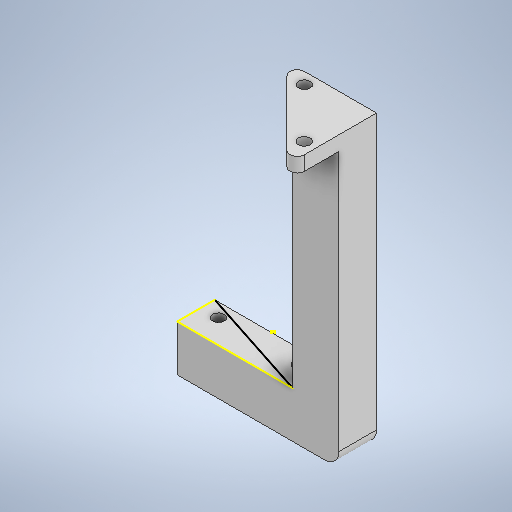
# Autodesk Inventor part: 13042026-12
Saved by Autodesk Inventor 2025.2 (Build 292293000, 293)
## iProperties
Created: 2026-05-05
Part Number: 13042026-12
Material: Generic
Document SubType Name: Modeling
Designer: Oski
Density: 1 g/cm^3
Appearance: Default
Author: Oski
Autodesk Inventor part; units mm, degrees
ref_plane "YZ Plane" through (0, 0, 0) normal (1, 0, 0) x (0, 1, 0)
ref_plane "XZ Plane" through (0, 0, 0) normal (0, 1, 0) x (-1, 0, 0)
ref_plane "XY Plane" through (0, 0, 0) normal (0, 0, 1) x (1, 0, 0)
sketch "Sketch2" plane through (0, 0, 0) normal (0, 0, 1) x (1, 0, 0)
  line L0 (-40, 16) -> (40, 16)
  line L1 (40, 16) -> (40, -16)
  line L2 (40, -16) -> (-40, -16)
  line L3 (-40, -16) -> (-40, 16)
  line L4 (-40, 16) -> (40, -16) construction
  line L5 (40, 16) -> (-40, -16) construction
  point P0 (0, 0)
  dimension "d4" = 32
  dimension "d5" = 80
  constraints: 12 end point, 2 midpoint, 2 parallel, 1 horizontal, 1 perpendicular
  measures "d4" distance of L0.end L1.end
  measures "d5" distance of L1.end L2.end
extrude "Extrusion1" add sketch "Sketch2" along normal blind 26
sketch "Sketch6" plane through (-40, 16, 0) normal (0, 1, 0) x (1, 0, 0)
  line L0 (12, -9.5) -> (0, -9.5) construction
  line L1 (0, 0) -> (0, -26) projected
  line L2 (68, -9.5) -> (80, -9.5) construction
  line L3 (80, 0) -> (80, -26) projected
  line L4 (80, 0) -> (0, 0) projected
  point P0 (40, 0)
  point P1 (74, -9.5)
  dimension "d29" = 56
  dimension "d30" = 9.5
  constraints: 4 end point, 3 point on line, 2 horizontal, 1 collinear, 1 midpoint
  measures "d29" distance of L2.start L0.start
  measures "d30" distance from line of L4 point (74, -9.5)
hole "Hole3" at (-28, 16, 9.5) at (28, 16, 9.5) direction (0, -1, 0) diameter 8.2 end through all
sketch "Sketch9" plane through (-40, 16, 0) normal (0, 1, 0) x (1, 0, 0)
  line L0 (0, 0) -> (0, -26) projected
  line L1 (80, -26) -> (0, -26) projected
  line L2 (0, 0) -> (80, -26)
  point P0 (40, 0)
  constraints: 2 end point
sketch "Sketch10" plane through (-40, 16, 0) normal (0, 1, 0) x (1, 0, 0)
  point P0 (40, 0)
sketch "Sketch11" plane through (40, -16, 0) normal (1, 0, 0) x (0, 0, -1)
  line L0 (0, 0) -> (0, 32) projected
  line L1 (0, 0) -> (-26, 0)
  line L2 (-26, 0) -> (-26, 200)
  line L3 (-26, 200) -> (0, 200)
  line L4 (0, 200) -> (0, 0)
  line L5 (-26, 0) -> (-26, 32) projected
  point P0 (0, 16)
  dimension "d52" = 200
  constraints: 8 end point, 2 parallel, 1 horizontal, 1 perpendicular, 1 point on line
  measures "d52" distance of L1.end L2.end
extrude "Extrusion4" add sketch "Sketch11" along normal blind 32
fillet "Fillet1" radius 10 1 edges at (72, -16, 13)
sketch "Sketch13" plane through (40, 184, 26) normal (0, 1, 0) x (1, 0, 0)
  line L0 (32, 26) -> (-30, 26)
  line L1 (0, 26) -> (-80, 26) projected
  line L2 (32, 26) -> (32, 0) projected
  line L3 (32, 26) -> (32, -36)
  line L4 (-30, 26) -> (32, -36)
  point P0 (-40, 26)
  dimension "d58" = 62
  constraints: 6 end point, 1 collinear, 1 perpendicular, 1 point on line
  measures "d58" distance of L0.start L0.end
extrude "Extrusion5" add sketch "Sketch13" against normal blind 10
fillet "Fillet2" radius 5 1 edges at (10, 179, 0)
fillet "Fillet3" radius 5 1 edges at (72, 179, 62)
sketch "Sketch15" plane through (22.0711, 184, 0) normal (0, 1, 0) x (1, 0, 0)
  line L0 (0, 0) -> (49.9289, 0) projected
  line L1 (49.9289, 0) -> (49.9289, -26) projected
  line L2 (49.9289, 0) -> (17.9289, 0)
  line L3 (17.9289, 0) -> (17.9289, -32)
  line L4 (17.9289, -32) -> (49.9289, -32)
  line L5 (49.9289, -32) -> (49.9289, 0)
  line L6 (49.9289, 0) -> (49.9289, -49.9289) projected
  point P0 (-22.0711, 0)
  point P1 (41.9289, -42)
  point P2 (7.9289, -8)
  dimension "d63" = 8
  dimension "d64" = 32
  dimension "d65" = 32
  dimension "d66" = 10
  dimension "d67" = 10
  dimension "d68" = 8
  constraints: 8 end point, 2 parallel, 1 horizontal, 1 perpendicular
  measures "d63" distance from line of L0 point (7.929, -8)
  measures "d64" distance of L3.end L4.end
  measures "d65" distance of L2.end L3.end
  measures "d66" distance from line of L3 point (7.929, -8)
  measures "d67" distance from line of L4 point (41.929, -42)
  measures "d68" distance from line of L6 point (41.929, -42)
hole "Hole6" at (30, 184, 8) at (64, 184, 42) direction (0, -1, 0) diameter 8.2 depth 20
body "Solid1"
